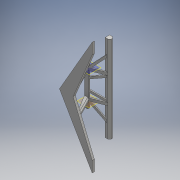
# Autodesk Inventor part: Spoiler_mk2
Saved by Autodesk Inventor 2016 (Build 200138000, 138)
## iProperties
Created: 2015-11-13
Part Number: Spoiler_mk2
Material: Generic
Document SubType Name: Modeling
Designer: Jared
Density: 1 g/cm^3
Appearance: Default
Author: Jared
Autodesk Inventor part; units mm, degrees
ref_plane "YZ Plane" through (0, 0, 0) normal (1, 0, 0) x (0, 1, 0)
ref_plane "XZ Plane" through (0, 0, 0) normal (0, 1, 0) x (-1, 0, 0)
ref_plane "XY Plane" through (0, 0, 0) normal (0, 0, 1) x (1, 0, 0)
sketch "Sketch1" plane through (0, 0, 0) normal (0, 1, 0) x (-1, 0, 0)
  circle A0 centre (0, 0) radius 1.4
  circle A1 centre (0, -73.1) radius 1.4
  arc A2 (4, 0) -> (-4, 0) centre (0, 0) ccw
  arc A3 (-4, -73.1) -> (4, -73.1) centre (0, -73.1) ccw
  line L0 (4, 0) -> (4, -73.1)
  line L1 (-4, -73.1) -> (-4, 0)
  dimension "d7" = 8
  dimension "d8" = 8
  constraints: 4 centre point, 4 end point, 4 point on circle, 2 coincident, 2 tangent
  measures "d7" diameter of A2
  measures "d8" diameter of A3
extrude "Extrusion1" add sketch "Sketch1" along normal blind 2
ref_plane "Work Plane2" through (4, 0, -10) normal (0, 0, -1) x (-1, 0, 0)
sketch "Sketch3" plane through (4, 0, -10) normal (0, 0, -1) x (-1, 0, 0)
  line L0 (8, 2) -> (0, 2) projected
  line L1 (1, 2) -> (-20, 10)
  line L2 (-20, 10) -> (-25, 10)
  line L3 (-25, 10) -> (0, 0)
  line L4 (0, 0) -> (0, 2) projected
  line L5 (0, 0) -> (0, 2)
  line L6 (0, 2) -> (1, 2)
  dimension "d22" = 5
  constraints: 10 end point, 2 collinear, 1 horizontal, 1 point on line
  measures "d22" distance of L1.end L2.end
extrude "Extrusion3" add sketch "Sketch3" along normal blind 5
ref_plane "Work Plane1" through (4, 0, -63.1) normal (0, 0, 1) x (1, 0, 0)
sketch "Sketch4" plane through (4, 0, -63.1) normal (0, 0, 1) x (1, 0, 0)
  line L0 (20, 10) -> (25, 10) projected
  line L1 (0, 0) -> (2, 0) projected
  line L2 (25, 10) -> (0, 0)
  line L3 (25, 10) -> (0, 0) projected
  line L4 (0, 0) -> (0, 2) projected
  line L5 (0, 0) -> (0, 2)
  line L6 (0, 2) -> (-1.0658, 2)
  line L7 (0, 2) -> (-8, 2) projected
  line L8 (20, 10) -> (-1.0658, 2)
  line L9 (20, 10) -> (25, 10)
  point P0 (-4, 0)
  constraints: 10 end point, 2 collinear, 1 parallel, 1 point on line
extrude "Extrusion4" add sketch "Sketch4" along normal blind 5
sketch "Sketch5" plane through (24, 10, -10) normal (0, 1, 0) x (1, 0, 0)
  line L0 (0, 0) -> (0, 5) projected
  line L1 (0, 0) -> (0, -53)
  line L2 (0, -53) -> (8, -53)
  line L3 (0, 53.1) -> (-21.0658, 53.1) projected
  line L4 (0, 53.1) -> (0, 106.1)
  line L5 (0, 106.1) -> (8, 106.1)
  line L6 (8, 106.1) -> (8, -53)
  line L7 (0, 0) -> (0, 53.1)
  point P0 (-24, -10)
  dimension "d27" = 53
  dimension "d28" = 8
  dimension "d29" = 53
  constraints: 12 end point, 3 perpendicular, 2 vertical, 1 parallel
  measures "d27" distance of L0.start L1.end
  measures "d28" distance of L1.end L2.end
  measures "d29" distance of L3.start L4.end
extrude "Extrusion5" add sketch "Sketch5" along normal blind 8
sketch "Sketch6" plane through (4, 0, -15) normal (0.3713907, -0.9284767, 0) x (0.9284767, 0.3713907, 0)
  line L0 (25.2546, -101.1) -> (25.2546, 58) projected
  line L1 (-0.1857, 7.3143) -> (25.2546, 32.7559)
  line L2 (26.9258, 5) -> (0, 5) projected
  line L3 (2.5, 5) -> (25.2546, 27.7558)
  line L4 (25.2546, 32.7559) -> (25.2546, 27.7558)
  line L5 (-0.1857, 5) -> (-0.1857, 0) projected
  line L6 (2.5, 5) -> (-0.1857, 5)
  line L7 (-0.1857, 5) -> (-0.1857, 7.3143)
  line L8 (0, 15) -> (0, 5) projected
  line L9 (0, -48.1) -> (0, -58.1) projected
  line L10 (0, -50.6) -> (25.2546, -75.8532)
  line L11 (0, -48.1) -> (26.9258, -48.1) projected
  line L12 (2.4999, -48.1) -> (25.2546, -70.8535)
  line L13 (25.2546, -75.8532) -> (25.2546, -70.8535)
  line L14 (0, -50.6) -> (0, -48.1)
  line L15 (0, -48.1) -> (2.4999, -48.1)
  line L16 (26.9258, 0) -> (0, 0) projected
  line L17 (25, 0) -> (0, -9.1007)
  line L18 (0, 0) -> (0, -43.1) projected
  line L19 (0, -9.1007) -> (0, -13.1007)
  line L20 (0, -13.1007) -> (25.2546, -3.9088)
  line L21 (25.2546, -3.9088) -> (25, 0)
  line L22 (0, -43.1) -> (26.9258, -43.1) projected
  line L23 (25, -43.1) -> (0, -34.0007)
  line L24 (25, -43.1) -> (51.6044, -43.1) construction
  line L25 (0, -34.0007) -> (0, -30.0007)
  line L26 (0, -30.0007) -> (25.2546, -39.1927)
  line L27 (25.2546, -39.1927) -> (25, -43.1)
  point P0 (-3.7139, 15)
  dimension "d32" = 4
  dimension "d33" = 70
  dimension "d34" = 160
  dimension "d35" = 4
  constraints: 38 end point, 16 point on line, 4 collinear, 4 parallel, 1 equal length, 1 horizontal, 1 vertical
  measures "d32" distance of L17.end L19.end
  measures "d33" angle of L20 L19
  measures "d34" angle of L24 L23
  measures "d35" distance of L23.end L25.end
extrude "Extrusion6" add sketch "Sketch6" against normal blind 2 contours L10 L9 L11 L12 L0 | L27 L23 L18 L26 | L20 L18 L17 L21 | L3 L2 L8 L1 L0 | L8 L6 L7 L1
chamfer "Chamfer1" distance 3 angle 45 2 edges at (32, 10, -36.55) (32, 18, -36.55)
sketch "Sketch7" plane through (4, 0, -63.1) normal (0, 0, 1) x (1, 0, 0)
  line L0 (15, -30) -> (10, -30)
  line L1 (10, -30) -> (15, -30)
  line L2 (0, 0) -> (23.4483, 9.3793) projected
  line L3 (15, -30) -> (0, 0)
  line L4 (0, 0) -> (-8, 0) projected
  line L5 (0, 0) -> (-8, 0)
  line L6 (-8, 0) -> (10, -30)
  point P0 (-4, 0)
  dimension "d41" = 5
  constraints: 10 end point, 2 collinear, 1 horizontal
  measures "d41" distance of L0.start L0.end
extrude "Extrusion7" add sketch "Sketch7" along normal blind 5
sketch "Sketch8" plane through (4, 0, -10) normal (0, 0, -1) x (-1, 0, 0)
  line L0 (0, 0) -> (8, 0) projected
  line L1 (-10, -30) -> (-15, -30) projected
  line L2 (0, 0) -> (-15, -30)
  line L3 (-15, -30) -> (-10, -30)
  line L4 (8, 0) -> (-10, -30) projected
  line L5 (-10, -30) -> (8, 0)
  line L6 (8, 0) -> (0, 0)
  point P0 (4, 0)
  constraints: 8 end point, 3 collinear
extrude "Extrusion8" add sketch "Sketch8" along normal blind 5
sketch "Sketch9" plane through (14, -30, -63.1) normal (0, -1, 0) x (1, 0, 0)
  line L0 (-30, 26.55) -> (30, -77.373)
  line L1 (-30, 26.55) -> (90, 26.55) construction
  line L2 (-30, 26.55) -> (30, 130.473)
  line L3 (-30, 26.55) -> (90, 26.55) construction
  line L4 (30, 130.473) -> (30, 110.473)
  line L5 (30, -77.373) -> (30, -57.373)
  line L6 (-5, 26.55) -> (30, 110.473)
  line L7 (-5, 26.55) -> (30, -57.373)
  point P0 (-14, 63.1)
  dimension "d46" = 120
  dimension "d47" = 60
  dimension "d49" = 120
  dimension "d50" = 60
  dimension "d51" = 20
  dimension "d52" = 30
  dimension "d53" = 20
  constraints: 16 end point, 2 equal length, 2 horizontal, 2 vertical, 1 point on line
  measures "d46" distance of L0.start L0.end
  measures "d47" angle of L0 L1
  measures "d49" distance of L0.start L2.end
  measures "d50" angle of L3 L2
  measures "d51" distance of L2.end L4.end
  measures "d52" angle of L2 L4
  measures "d53" distance of L0.end L5.end
extrude "Extrusion9" add sketch "Sketch9" along normal blind 4
chamfer "Chamfer2" distance 2 angle 45 2 edges at (11.5, -15, -58.1) (11.5, -15, -15)
body "Solid1"
